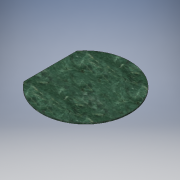
# Autodesk Inventor part: CortexPCB
Saved by Autodesk Inventor 2018 (Build 220112000, 112)
## iProperties
Created: 2017-06-11
Part Number: CortexPCB
Material: Generisch
Document SubType Name: Modeling
Designer: JochenAlt
Density: 1 g/cm^3
Appearance: Grün - poliert
Author: JochenAlt
Autodesk Inventor part; units mm, degrees
ref_plane "YZ Plane" through (0, 0, 0) normal (1, 0, 0) x (0, 1, 0)
ref_plane "XZ Plane" through (0, 0, 0) normal (0, 1, 0) x (-1, 0, 0)
ref_plane "XY Plane" through (0, 0, 0) normal (0, 0, 1) x (1, 0, 0)
sketch "Skizze1" plane through (0, 0, 0) normal (0, 0, 1) x (1, 0, 0)
  line L0 (-70.7, 0) -> (70.7, 0) construction
  arc A0 (-40.5, -30.1662) -> (-40.5, 30.1662) centre (0, 0) ccw
  line L1 (-40.5, 30.1662) -> (-40.5, -30.1662)
  line L2 (40.5, 30.1662) -> (-40.5, -30.1662) construction
  line L3 (-40.5, 30.1662) -> (40.5, -30.1662) construction
  point P0 (0, 48)
  point P1 (0, -48)
  point P2 (-50.5, 0)
  dimension "d3" = 96
  dimension "d15" = 50.5
  dimension "d17" = 10
  dimension "d19" = 30.1662
  constraints: 7 end point, 2 midpoint, 2 point on circle, 1 centre point, 1 coincident, 1 point on line, 1 symmetric about line
  measures "d3" distance of point (0, -48) point (0, 48)
  measures "d15" distance of point (-50.5, 0) point (0, 0)
  measures "d17" distance from line of L1 point (-50.5, 0)
  measures "d19" distance from line of L1.end L0
extrude "Extrusion1" add sketch "Skizze1" along normal blind 1.5
hole "Bohrung1" at (0, 48, 0) at (0, -48, 0) direction (0, 0, 1) diameter 2.1 end through all
